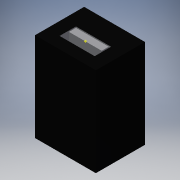
# Autodesk Inventor part: usbRangeExtender
Saved by Autodesk Inventor 2016 (Build 200138000, 138)
## iProperties
Created: 2015-10-17
Part Number: usbRangeExtender
Material: Generic
Document SubType Name: Modeling
Designer: Artur
Density: 1 g/cm^3
Appearance: Default
Mass: 18.228 g
Surface Area: 64.94 cm^2
Volume: 18.228 cm^3
Author: Artur
Autodesk Inventor part; units mm, degrees
ref_plane "YZ Plane" through (0, 0, 0) normal (1, 0, 0) x (0, 1, 0)
ref_plane "XZ Plane" through (0, 0, 0) normal (0, 1, 0) x (-1, 0, 0)
ref_plane "XY Plane" through (0, 0, 0) normal (0, 0, 1) x (1, 0, 0)
sketch "Sketch1" plane through (0, 0, 0) normal (0, 1, 0) x (-1, 0, 0)
  line L0 (26, 0) -> (0, 0)
  line L1 (0, 0) -> (0, -38)
  line L2 (0, -38) -> (26, -38)
  line L3 (26, -38) -> (26, 0)
  dimension "d0" = 38
  dimension "d1" = 26
  constraints: 8 end point, 2 parallel, 1 coincident, 1 horizontal, 1 perpendicular
  measures "d0" distance of L2.end L0.start
  measures "d1" distance of L1.end L2.end
extrude "Extrusion1" add sketch "Sketch1" along normal blind 21
sketch "Sketch2" plane through (0, 21, 0) normal (0, 1, 0) x (1, 0, 0)
  line L0 (-19.5, 30) -> (-6.5, 30)
  line L1 (0, 38) -> (-26, 38) projected
  line L2 (-26, 38) -> (-26, 0) projected
  line L3 (-6.5, 30) -> (-6.5, 23)
  line L4 (-13, 30) -> (-13, 10.7779) construction
  line L5 (-16.5, 21) -> (-9.5, 21)
  line L6 (-6.5, 23) -> (-9.5, 23)
  line L7 (-9.5, 23) -> (-9.5, 21)
  line L8 (-16.5, 21) -> (-16.5, 23)
  line L9 (-16.5, 23) -> (-19.5, 23)
  line L10 (-19.5, 23) -> (-19.5, 30)
  point P0 (0, 0)
  point P1 (-13, 21)
  point P2 (-13, 26.5)
  dimension "d4" = 8
  dimension "d5" = 13
  dimension "d6" = 26
  dimension "d7" = 6.5
  dimension "d8" = 7
  dimension "d9" = 7
  dimension "d10" = 2
  constraints: 18 end point, 3 perpendicular, 3 point on line, 3 vertical, 2 horizontal, 2 midpoint, 1 parallel
  measures "d4" distance between parallel lines of L0 L1
  measures "d5" distance of L0.start L0.end
  measures "d6" distance of L1.start L1.end
  measures "d7" distance from line of L2 L0.start
  measures "d8" distance of L0.end L3.end
  measures "d9" distance of L5.start L5.end
  measures "d10" vertical distance of L5.end L3.end
extrude "Extrusion2" cut sketch "Sketch2" against normal blind 15
sketch "Sketch3" plane through (-26, 0, 0) normal (0, 0, 1) x (1, 0, 0)
  line L0 (5.5, 5) -> (20.5, 5)
  line L1 (0, 0) -> (26, 0) projected
  line L2 (13, 0) -> (13, 33.23) construction
  line L3 (5.5, 5) -> (5.5, 12)
  line L4 (5.5, 12) -> (20.5, 12)
  line L5 (20.5, 12) -> (20.5, 5)
  line L6 (6, 11.5) -> (20, 11.5)
  line L7 (20, 11.5) -> (20, 8.5)
  line L8 (20, 8.5) -> (6, 8.5)
  line L9 (6, 8.5) -> (6, 11.5)
  point P0 (13, 5)
  point P1 (13, 8.5)
  dimension "d13" = 5
  dimension "d14" = 15
  dimension "d15" = 7
  dimension "d16" = 14
  dimension "d17" = 3
  dimension "d18" = 0.5
  dimension "d19" = 0.5
  constraints: 18 end point, 3 midpoint, 3 perpendicular, 2 horizontal, 2 parallel, 2 vertical, 1 point on line
  measures "d13" distance between parallel lines of L1 L0
  measures "d14" distance of L0.start L0.end
  measures "d15" distance of L0.start L3.end
  measures "d16" distance of L6.start L6.end
  measures "d17" distance of L8.end L6.start
  measures "d18" distance between parallel lines of L3 L9
  measures "d19" distance between parallel lines of L4 L6
extrude "Extrusion3" cut sketch "Sketch3" against normal blind 15
equation "\"d7\" = -0.5 * d5 + 0.5 * d6"
body "Solid1"
